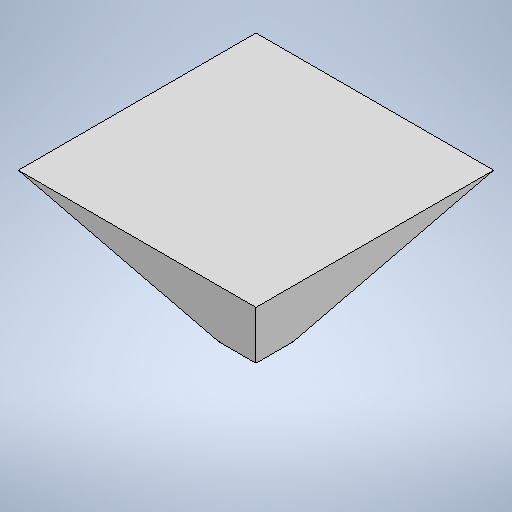
# Autodesk Inventor part: NDM-VOS dummy2
Saved by Autodesk Inventor 2025 (Build 290162010, 162A)
## iProperties
Created: 2024-07-24
Part Number: NDM-VOS dummy2
Material: Water
Document SubType Name: Modeling
Designer: admin
Mass: 2.28943e+06 g
Surface Area: 138396 cm^2
Volume: 2.29333e+06 cm^3
Density: 0.9983 g/cm^3
Appearance: Default
Author: admin
Autodesk Inventor part; units mm, degrees
ref_plane "YZ Plane" through (0, 0, 0) normal (1, 0, 0) x (0, 1, 0)
ref_plane "XZ Plane" through (0, 0, 0) normal (0, 1, 0) x (-1, 0, 0)
ref_plane "XY Plane" through (0, 0, 0) normal (0, 0, 1) x (1, 0, 0)
sketch "Sketch1" plane through (0, 0, 0) normal (0, 0, 1) x (1, 0, 0)
  line L0 (-125, 125) -> (125, 125)
  line L1 (125, 125) -> (125, -125)
  line L2 (125, -125) -> (-125, -125)
  line L3 (-125, -125) -> (-125, 125)
  line L4 (-125, 125) -> (125, -125) construction
  line L5 (125, 125) -> (-125, -125) construction
  point P0 (0, 0)
  dimension "d0" = 250
  dimension "d1" = 250
  constraints: 12 end point, 2 midpoint, 2 parallel, 1 horizontal, 1 perpendicular
  measures "d0" distance of L1.end L2.end
  measures "d1" distance of L0.end L1.end
extrude "Extrusion1" add sketch "Sketch1" along normal blind 1000 draft 34
body "Solid1"
